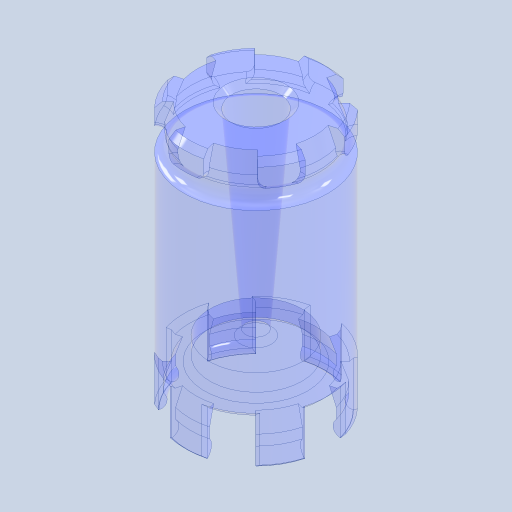
# Autodesk Inventor part: cpd_ultra-TLA100.3_0.7_p3_20230615
Saved by Autodesk Inventor 2024 (Build 280153000, 153)
## iProperties
Created: 2022-02-17
Part Number: cpd_ultra-TLA100.3_0.7_p3_20230615
Material: Generic
Document SubType Name: Modeling
Designer: to172
Density: 1 g/cm^3
Appearance: Clear - Blue
Author: to172
Autodesk Inventor part; units mm, degrees
ref_plane "YZ Plane" through (0, 0, 0) normal (1, 0, 0) x (0, 1, 0)
ref_plane "XZ Plane" through (0, 0, 0) normal (0, 1, 0) x (-1, 0, 0)
ref_plane "XY Plane" through (0, 0, 0) normal (0, 0, 1) x (1, 0, 0)
sketch "Sketch1" plane through (0, 0, 0) normal (0, 0, 1) x (1, 0, 0)
  line L0 (0, 0) -> (14.95, 0) construction
  line L1 (0, 0) -> (0, 13.4) construction
  line L2 (0.7264, 0) -> (2.2126, 20)
  line L3 (2.2126, 20) -> (6.4, 20)
  line L4 (6.4, 20) -> (6.4, 0)
  line L5 (6.4, 0) -> (0.7264, 0)
  line L6 (0, 0) -> (4.1, 0)
  line L7 (4.1, 0) -> (4.1, 2)
  line L8 (4.1, 2) -> (0.875, 2)
  dimension "d0" = 4.25
  dimension "d2" = 6.4
  dimension "d3" = 20
  dimension "d16" = 0.875
  dimension "d17" = 4.1
  dimension "d18" = 2
  constraints: 18 end point, 3 horizontal, 3 perpendicular, 3 point on line, 1 collinear, 1 parallel, 1 vertical
  measures "d0" angle of L2 L1
  measures "d2" distance between parallel lines of L4 L1
  measures "d3" distance between parallel lines of L0 L3
  measures "d16" distance from line of L1 L8.end
  measures "d17" distance between parallel lines of L7 L1
  measures "d18" distance between parallel lines of L8 L0
revolve "Revolution1" add sketch "Sketch1" angle 360 about axis through (0, 0, 0) along (0, 1, 0) contours L2 L3 L4 L5 L7 L8
sketch "Sketch2" plane through (0, 0, 0) normal (1, 0, 0) x (0, 1, 0)
  line L0 (0, 0.1182) -> (0, -10.17) construction
  line L1 (0, -6.4) -> (-3.75, -6.4)
  line L2 (-3.75, -6.4) -> (-3.75, -5.85)
  line L3 (-3.75, -5.85) -> (0, -5.85)
  line L4 (0, -5.85) -> (0, -6.4)
  line L5 (0, 6.4) -> (0, -6.4) construction
  line L6 (20, -6.4) -> (0, -6.4) construction
  line L7 (-10.5292, 0) -> (25.0882, 0) projected
  circle A0 centre (-3, -6.4) radius 0.8
  line L8 (-1.5, -5.85) -> (0, -5.35)
  line L9 (0, -5.35) -> (0, -5.85)
  point P0 (0, 0)
  point P1 (-5.441, -6)
  point P2 (-2.4191, -5.85)
  point P3 (-3.75, -6.1216)
  dimension "d5" = 0.55
  dimension "d37" = 3.75
  dimension "d38" = 1.6
  dimension "d39" = 0.75
  dimension "d40" = 1.5
  dimension "d41" = 0.5
  constraints: 14 end point, 4 collinear, 3 point on line, 2 parallel, 1 centre point, 1 horizontal, 1 perpendicular, 1 vertical
  measures "d5" distance between parallel lines of L1 L3
  measures "d37" distance between parallel lines of L0 L2
  measures "d38" diameter of A0
  measures "d39" distance from line of A0.centre L2
  measures "d40" distance from line of L0 L8.start
  measures "d41" distance from line of L3 L8.end
revolve "Revolution2" add sketch "Sketch2" angle 30 mid plane about axis through (0, -10, 0) along (0, 1, 0) contours L1 A0 L3 L4 | L1 L2 A0 L3 | L3 L8 L9 | L3 A0
chamfer "Chamfer1" distance 0.25 angle 45 3 edges at (-1.6564, -1.875, -6.1819) (1.6564, -1.875, -6.1819) (0, -3.75, -6.4)
pattern_circular "Circular Pattern1" count 6 over 360 about axis through (0, -10, 0) along (0, 1, 0) of "Revolution2", "Chamfer1"
chamfer "Chamfer2" distance 0.5 angle 45 18 edges at (-4.613, 0, 4.4362) (-3.2, 0, 5.5426) (-1.5354, 0, 6.2131) (-4.1, 0, 0) (-6.1484, 0, -1.7769) (-6.4, 0, 0) (-6.1484, 0, 1.7769) (-3.0911, 0, -5.604) (-4.613, 0, -4.4362) (4.613, 0, -4.4362) (3.0911, 0, -5.604) (6.1484, 0, -1.7769) (6.3452, 0, -0.8354) (6.3452, 0, 0.8354) (6.1484, 0, 1.7769) (4.613, 0, 4.4362) (3.2, 0, 5.5426) (1.5354, 0, 6.2131)
sketch "Sketch3" plane through (0, 0, 0) normal (0, 0, 1) x (0, 1, 0)
  line L0 (0, 0) -> (0, -9.9283) construction
  line L1 (0, 4.1) -> (0, -4.1) construction
  line L2 (0, 0) -> (10.6094, 0) construction
  line L3 (20, 4) -> (20, -4) construction
  line L4 (20, 0) -> (20, -8.6257) construction
  circle A0 centre (17, -6.4) radius 0.85
  line L5 (20, -6.4) -> (17, -6.4)
  line L6 (17, -6.4) -> (20, -6.4)
  line L7 (20, -6.4) -> (20, -5.75)
  line L8 (20, -5.75) -> (17, -5.75)
  line L9 (17, -5.75) -> (17, -6.4)
  line L10 (20, 6.4) -> (20, -6.4) projected
  line L11 (0.5, -1.4137) -> (-3.5, -1.4137) projected
  line L12 (0.5, -4.6988) -> (0.5, -1.4137) projected
  line L13 (-3.5, -4.6988) -> (0.5, -4.6988) projected
  line L14 (-3.5, -6.1125) -> (-3.5, -4.6988) projected
  line L15 (0.5, -6.1125) -> (-3.5, -6.1125) projected
  line L16 (0.5, -6.1125) -> (0.5, -6.1125) projected
  line L17 (-3.5, -6.1125) -> (0.5, -6.1125) projected
  line L18 (-3.5, -4.6988) -> (-3.5, -6.1125) projected
  line L19 (0.5, -4.6988) -> (-3.5, -4.6988) projected
  line L20 (0.5, -1.4137) -> (0.5, -4.6988) projected
  line L21 (-3.5, -1.4137) -> (0.5, -1.4137) projected
  line L22 (-3.5, 1.4137) -> (-3.5, -1.4137) projected
  line L23 (0.5, 1.4137) -> (-3.5, 1.4137) projected
  line L24 (0.5, 4.6988) -> (0.5, 1.4137) projected
  line L25 (-3.5, 4.6988) -> (0.5, 4.6988) projected
  line L26 (-3.5, 6.1125) -> (-3.5, 4.6988) projected
  line L27 (0.5, 6.1125) -> (-3.5, 6.1125) projected
  line L28 (0.5, 6.1125) -> (0.5, 6.1125) projected
  line L29 (-3.5, 6.1125) -> (0.5, 6.1125) projected
  line L30 (-3.5, 4.6988) -> (-3.5, 6.1125) projected
  line L31 (0.5, 4.6988) -> (-3.5, 4.6988) projected
  line L32 (0.5, 1.4137) -> (0.5, 4.6988) projected
  line L33 (-3.5, 1.4137) -> (0.5, 1.4137) projected
  line L34 (-3.5, -1.4137) -> (-3.5, 1.4137) projected
  line L35 (20, 6.4) -> (20, -6.4) projected
  line L36 (20, -6.4) -> (0.5, -6.4) projected
  line L37 (-8.2, 0) -> (24.7, 0) projected
  line L38 (18.45, -5.75) -> (20, -5.2)
  line L39 (20, -5.2) -> (20, -5.75)
  point P0 (-1.5, -6.5)
  point P1 (0, -6.5)
  point P2 (1.75, -6.5)
  point P3 (2.25, -6.5)
  point P4 (17.85, -6.4)
  point P5 (16.15, -6.4)
  point P6 (17.5477, -5.75)
  point P7 (20, -5.75)
  dimension "d22" = 1.7
  dimension "d23" = 3
  dimension "d24" = 0.65
  dimension "d42" = 0.55
  dimension "d43" = 1.55
  constraints: 24 end point, 5 collinear, 4 point on line, 2 horizontal, 2 parallel, 1 centre point, 1 midpoint, 1 perpendicular
  measures "d22" diameter of A0
  measures "d23" distance between parallel lines of L4 L9
  measures "d24" distance between parallel lines of L8 L5
  measures "d42" distance from line of L8 L38.end
  measures "d43" distance from line of L4 L38.start
revolve "Revolution3" cut sketch "Sketch3" angle 360 about axis through (0, -10, 0) along (0, 1, 0) contours L5 L9 L8 A0 | L8 L9 L36 A0
revolve "Revolution4" cut sketch "Sketch3" angle 32 mid plane about axis through (0, -10, 0) along (0, 1, 0) contours A0 L8 L7 L5 | L38 L10 L8
fillet "Fillet1" radius 0.5 4 edges at (5.694, 17.5477, 0.8002) (5.694, 17.5477, -0.8002) (5.8075, 17.7707, 1.6653) (5.8075, 17.7707, -1.6653)
pattern_circular "Circular Pattern2" count 6 over 360 about axis through (0, -10, 0) along (0, 1, 0) of "Revolution4", "Fillet1"
chamfer "Chamfer3" distance 0.5 angle 45 8 edges at (5.5426, 20, 3.2) (0, 20, 6.4) (-5.5426, 20, 3.2) (-5.5426, 20, -3.2) (0, 20, -6.4) (5.5426, 20, -3.2) (-2.2126, 20, 0) (-0.875, 2, 0)
body "Solid1"
